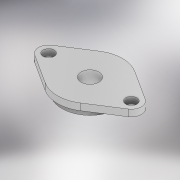
# Autodesk Inventor part: screw_bracket
Saved by Autodesk Inventor 2020 (Build 240168000, 168)
## iProperties
Created: 2020-06-18
Part Number: screw_bracket
Material: Generic
Document SubType Name: Modeling
Designer: pc-konvi
Density: 1 g/cm^3
Appearance: Default
Author: pc-konvi
Autodesk Inventor part; units mm, degrees
ref_plane "YZ Plane" through (0, 0, 0) normal (1, 0, 0) x (0, 1, 0)
ref_plane "XZ Plane" through (0, 0, 0) normal (0, 1, 0) x (-1, 0, 0)
ref_plane "XY Plane" through (0, 0, 0) normal (0, 0, 1) x (1, 0, 0)
sketch "Sketch1" plane through (0, 0, 0) normal (0, 1, 0) x (-1, 0, 0)
  circle A0 centre (0, 0) radius 4
  circle A1 centre (0, 0) radius 6
  dimension "d0" = 8
  dimension "d1" = 2
  constraints: 2 centre point, 1 coincident
  measures "d0" diameter of A0
  measures "d1" radial gap between concentric circles of A0 A1
extrude "Extrusion1" add sketch "Sketch1" along normal blind 4
sketch "Sketch2" plane through (0, 4, 0) normal (0, 1, 0) x (1, 0, 0)
  circle A0 centre (0, 0) radius 12.5
  circle A1 centre (0, 0) radius 4 projected
  dimension "d4" = 25
  constraints: 1 centre point, 1 coincident
  measures "d4" diameter of A0
extrude "Extrusion2" add sketch "Sketch2" along normal blind 3
sketch "Sketch3" plane through (0, 7, 0) normal (0, 1, 0) x (1, 0, 0)
  circle A0 centre (-18.5, 0) radius 2.5
  circle A1 centre (18.5, 0) radius 2.5
  circle A2 centre (0, 0) radius 12.5 construction
  circle A3 centre (0, 0) radius 14.5
  circle A4 centre (-18.5, 0) radius 4.5
  circle A5 centre (18.5, 0) radius 4.5
  line L0 (-20.9324, 3.7859) -> (-7.8378, 12.1991)
  line L1 (-20.9324, -3.7859) -> (-7.8378, -12.1991)
  line L2 (20.9324, 3.7859) -> (7.8378, 12.1991)
  line L3 (20.9324, -3.7859) -> (7.8378, -12.1991)
  circle A6 centre (0, 0) radius 4 projected
  point P0 (-14.3851, -1.8215)
  point P1 (-14.3851, 1.8215)
  point P2 (14.3851, 1.8215)
  point P3 (14.3851, -1.8215)
  dimension "d7" = 5
  dimension "d8" = 5
  dimension "d9" = 37
  dimension "d10" = 18.5
  dimension "d11" = 2
  dimension "d12" = 2
  dimension "d13" = 2
  constraints: 8 end point, 8 point on circle, 8 tangent, 5 centre point, 2 horizontal alignment
  measures "d7" diameter of A0
  measures "d8" diameter of A1
  measures "d9" distance of A1.centre A0.centre
  measures "d10" distance of point (0, 0) A1.centre
  measures "d11" radial gap between concentric circles of A2 A3
  measures "d12" radial gap between concentric circles of A0 A4
  measures "d13" radial gap between concentric circles of A1 A5
extrude "Extrusion3" add sketch "Sketch3" along normal blind 3
equation "\"d10\" = 0.5 * d9"
body "Solid1"
